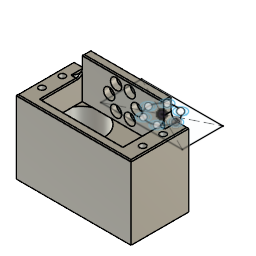
Down Bracket v2 (Autodesk Fusion 360 design; units mm, degrees)
Autodesk Fusion 360 part; units mm, degrees
sketch "Sketch1" plane through (0, 0, 0) normal (0, 0, 1) x (1, 0, 0)
  circle A0 centre (0, 0) radius 6.725
  circle A1 centre (6.725, 0) radius 1.65
  circle A2 centre (3.3625, 5.824) radius 1.65
  circle A3 centre (-3.3625, 5.824) radius 1.65
  circle A4 centre (-6.725, 0) radius 1.65
  circle A5 centre (-3.3625, -5.824) radius 1.65
  circle A6 centre (3.3625, -5.824) radius 1.65
  circle A7 centre (6.725, 0) radius 2.75
  circle A8 centre (3.3625, 5.824) radius 2.75
  circle A9 centre (-3.3625, 5.824) radius 2.75
  circle A10 centre (-6.725, 0) radius 2.75
  circle A11 centre (-3.3625, -5.824) radius 2.75
  circle A12 centre (3.3625, -5.824) radius 2.75
  line L0 (20, -10) -> (-20, -10)
  line L1 (-20, -10) -> (-20, 10)
  line L2 (-20, 10) -> (20, 10)
  line L3 (20, 10) -> (20, -10)
  line L4 (20, -10) -> (-20, 10) construction
  line L5 (-20, -10) -> (20, 10) construction
  dimension "d1" = 13.45
  dimension "d2" = 3.3
  dimension "d4" = 360
  dimension "d5" = 5.5
  dimension "d7" = 360
  dimension "d8" = 40
  dimension "d9" = 20
  constraint coincident A0.centre origin
  constraint coincident A0 A1.centre
  constraint concentric A1 A7
  constraint horizontal L0
  constraint perpendicular L0 L1
  constraint parallel L0 L2
  constraint parallel L1 L3
  constraint coincident L4 A0.centre
  constraint coincident L5 A0.centre
  measures "d1" diameter of A0
  measures "d2" diameter of A1
  measures "d5" diameter of A7
  measures "d8" distance of L1.end L2.end
  measures "d9" distance of L0.end L1.end
extrude "Extrude1" add sketch "Sketch1" along normal blind 4.2 contours A0 A7 A8 A9 A10 A11 A12 | L0 L1 L2 L3 makes body 1
extrude "Extrude2" add sketch "Sketch1" along normal blind 1.2 separate body contours A0 A1 A7 | A0 A1 A7 | A0 A2 A8 | A0 A2 A8 | A0 A6 A12 | A0 A6 A12 | A0 A3 A9 | A0 A3 A9 | A0 A5 A11 | A0 A5 A11 | A0 A4 A10 | A0 A4 A10 makes body 2 at (6.0988, -6.0978, 0.4) makes body 3 at (-0.6262, 5.5502, 0.4) makes body 4 at (-0.6262, -6.0978, 0.4) makes body 5 at (9.4613, -0.2738, 0.4) makes body 6 at (6.0988, 5.5502, 0.4) makes body 7 at (-3.9887, -0.2738, 0.4)
sketch "Sketch2" plane through (0, -10, 0) normal (0, -1, 0) x (1, 0, 0)
  line L0 (-20, 0) -> (20, 0)
  line L1 (20, 0) -> (20, 4.2)
  line L2 (20, 4.2) -> (-20, 4.2)
  line L3 (-20, 4.2) -> (-20, 0)
  line L4 (-20, 4.2) -> (20, 4.2)
  line L5 (20, 4.2) -> (20, 24.2)
  line L6 (20, 24.2) -> (-20, 24.2)
  line L7 (-20, 24.2) -> (-20, 4.2)
  line L8 (20, 0) -> (-20, 0)
  line L9 (0, 24.2) -> (0, 4.2) construction
  line L10 (24.2, 0) -> (-24.2, 0)
  line L11 (-24.2, 0) -> (-24.2, 28.4)
  line L12 (-24.2, 28.4) -> (24.2, 28.4)
  line L13 (24.2, 28.4) -> (24.2, 0)
  line L14 (24.2, 0) -> (-24.2, 28.4) construction
  line L15 (-24.2, 0) -> (24.2, 28.4) construction
  point P0 (0, 14.2)
  dimension "d14" = 20
  dimension "d15" = 4.2
  constraint horizontal L4
  constraint vertical L5
  constraint horizontal L6
  constraint vertical L7
  constraint coincident L2.end L3.start
  constraint midpoint L6 L9.start
  constraint midpoint L4 L9.end
  constraint horizontal L10
  constraint perpendicular L10 L11
  constraint parallel L10 L12
  constraint parallel L11 L13
  constraint coincident L14 P0
  constraint coincident L15 P0
  constraint midpoint L9 P0
  measures "d14" distance of L2.end L6.end
  measures "d15" distance of L4 L8
extrude "Extrude3" add sketch "Sketch2" against normal blind 11 contours L1 L3 L5 L6 L7 L10 L11 L12 L13 bodies 1
sketch "Sketch3" plane through (0, -10, 0) normal (0, -1, 0) x (1, 0, 0)
  line L0 (-24.2, 0) -> (24.2, 0)
  line L1 (24.2, 0) -> (24.2, 28.4)
  line L2 (24.2, 28.4) -> (-24.2, 28.4)
  line L3 (-24.2, 28.4) -> (-24.2, 0)
  line L4 (-20, 4.2) -> (-20, 24.2)
  line L5 (-20, 24.2) -> (20, 24.2)
  line L6 (20, 24.2) -> (20, 4.2)
  line L7 (20, 4.2) -> (-20, 4.2)
  line L8 (20, 4.2) -> (20, 24.2) construction
  line L9 (20, 14.2) -> (-10.4, 14.2) construction
  circle A0 centre (-10.4, 14.2) radius 11
  line L10 (-20, 14.2) -> (-10.4, 14.2)
  dimension "d19" = 30.4
  dimension "d20" = 22
  dimension "d40" = 9.6
  constraint coincident L6.end L7.start
  constraint coincident L5.end L6.start
  constraint midpoint L6 L9.start
  constraint perpendicular L6 L9
  constraint coincident L9.end A0.centre
  constraint midpoint L4 L10.start
  constraint perpendicular L4 L10
  measures "d19" distance of L9.start L9.end
  measures "d20" diameter of A0
  measures "d40" distance of L10.start L9.end
extrude "Extrude4" add sketch "Sketch3" along normal blind 5 contours L0 L1 L2 L3 | L4 L7 A0 | L4 L5 A0 | L5 L6 L7 A0 bodies 1
move_body "Move1" bodies 1 3 4 2 6 7 5 to x (1, 0, 0) y (0, 0, 1) z (0, -1, 0) at (0, -15, 15)
sketch "Sketch4" plane through (0, 0, 16) normal (0, 0, 1) x (-1, 0, 0)
  line L0 (24.2, 43.4) -> (-24.2, 43.4)
  line L1 (-24.2, 43.4) -> (-24.2, 15)
  line L2 (-24.2, 15) -> (-20, 15)
  line L3 (-20, 15) -> (-20, 19.2)
  line L4 (-20, 19.2) -> (-20, 39.2)
  line L5 (-20, 39.2) -> (20, 39.2)
  line L6 (20, 39.2) -> (20, 19.2)
  line L7 (20, 19.2) -> (20, 15)
  line L8 (20, 15) -> (24.2, 15)
  line L9 (24.2, 15) -> (24.2, 43.4)
  line L10 (20, 19.2) -> (20, 39.2)
  line L11 (24.75, 29.2) -> (24.75, 34.2)
  circle A0 centre (24.75, 34.2) radius 1.525
  line L12 (-20, 19.2) -> (20, 19.2) construction
  line L13 (0, 39.2) -> (0, 19.2) construction
  line L14 (0, 29.2) -> (20, 29.2) construction
  circle A1 centre (24.75, 24.2) radius 1.525
  circle A2 centre (-24.75, 34.2) radius 1.525
  circle A3 centre (-24.75, 24.2) radius 1.525
  dimension "d23" = 5
  dimension "d24" = 3.05
  dimension "d25" = 10
  dimension "d26" = 49.5
  constraint coincident L6.end L7.start
  constraint coincident L5.end L6.start
  constraint coincident L11.end A0.centre
  constraint midpoint L5 L13.start
  constraint midpoint L12 L13.end
  constraint coincident L13 L14.start
  constraint coincident L10 L14.end
  constraint perpendicular L10 L14
  constraint symmetric A0 L14 A1
  constraint symmetric A0 L13 A2
  constraint symmetric L13 A1 A3
  measures "d23" distance of L11.start L11.end
  measures "d24" diameter of A0
  measures "d25" distance of L11.end A1.centre
  measures "d26" distance of L11.end A2.centre
extrude "Extrude5" add 1 faces at (24.2, -33.9333, 5.3333) along direction (1, 0, 0) blind 4 on bodies 1 bodies 1
extrude "Extrude6" add 1 faces at (-24.2, -24.4667, 5.3333) along direction (-1, 0, 0) blind 4 on bodies 1 bodies 1
extrude "Extrude7" cut sketch "Sketch4" against normal blind 10 contours L9 A0 | L9 A0 | L1 A2 | L1 A2 | L9 A1 | L9 A1 | L1 A3 | L1 A3 bodies 1
fillet "Fillet1" radius 3 2 edges at (-20, -17.1, 16) (20, -17.1, 16) on bodies 1
fillet "Fillet2" radius 2.5 2 edges at (21.5, -19.2, 16) (-21.5, -19.2, 16) on bodies 1
fillet "Fillet3" radius 0.5 18 edges at (20, -17.1, 25) (0, -15, 25) (0, -19.2, 25) (-20, -17.1, 25) (-20, -15, 22) (-20.8787, -15, 16.8787) (-25.6, -15, 16) (-28.2, -29.2, 16) (0, -43.4, 16) (28.2, -29.2, 16) (-20, -30.45, 16) (-20, -19.9322, 16.7322) (0, -39.2, 16) (20, -19.9322, 16.7322) (20, -30.45, 16) (20, -15, 22) (20.8787, -15, 16.8787) (25.6, -15, 16) on bodies 1
extrude "Extrude8" add 1 faces at (19, -29.2, 0) along direction (0, 0, -1) blind 20 on bodies 1 bodies 1
equation "d19 = 40 mm - 9.6 mm"
